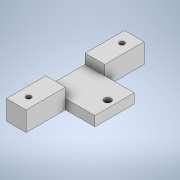
# Autodesk Inventor part: clawstack
Saved by Autodesk Inventor 2020 (Build 240168000, 168)
## iProperties
Created: 2020-03-11
Part Number: clawstack
Material: Generic
Document SubType Name: Modeling
Designer: cs1874
Density: 1 g/cm^3
Appearance: Default
Author: cs1874
Autodesk Inventor part; units mm, degrees
ref_plane "YZ Plane" through (0, 0, 0) normal (1, 0, 0) x (0, 1, 0)
ref_plane "XZ Plane" through (0, 0, 0) normal (0, 1, 0) x (-1, 0, 0)
ref_plane "XY Plane" through (0, 0, 0) normal (0, 0, 1) x (1, 0, 0)
sketch "Sketch1" plane through (0, 0, 0) normal (0, 1, 0) x (-1, 0, 0)
  line L0 (0, 0) -> (10, 0)
  line L1 (10, 0) -> (10, -60)
  line L2 (10, -60) -> (0, -60)
  line L3 (0, -60) -> (0, 0)
  line L4 (5, 0) -> (5, -6.25)
  circle A0 centre (5, -6.25) radius 1.3
  line L5 (5, -60) -> (5, -53.75)
  circle A1 centre (5, -53.75) radius 1.3
  dimension "d0" = 10
  dimension "d1" = 60
  dimension "d2" = 6.25
  dimension "d3" = 2.6
  dimension "d4" = 6.25
  dimension "d5" = 2.6
  constraints: 12 end point, 2 centre point, 2 coincident, 2 midpoint, 2 parallel, 2 vertical, 1 horizontal, 1 perpendicular
  measures "d0" distance of L1.end L2.end
  measures "d1" distance of L0.end L1.end
  measures "d2" distance of L4.start L4.end
  measures "d3" diameter of A0
  measures "d4" distance of L5.start L5.end
  measures "d5" diameter of A1
extrude "Extrusion1" add sketch "Sketch1" along normal blind 10
sketch "Sketch4" plane through (0, 10, 0) normal (0, 1, 0) x (1, 0, 0)
  line L0 (0, 0) -> (0, 60) projected
  line L1 (0, 0) -> (0, 10)
  line L2 (0, 60) -> (0, 40)
  line L3 (-10, 60) -> (-10, 0) projected
  line L4 (-10, 10) -> (-10, 50)
  line L5 (0, 50) -> (0, 10)
  line L6 (-10, 0) -> (0, 0) projected
  line L7 (0, 0) -> (0, 20)
  line L8 (0, 20) -> (-10, 20)
  line L9 (-10, 60) -> (-10, 40)
  line L10 (-10, 60) -> (10, 60) construction
  line L11 (-10, 40) -> (0, 40)
  dimension "d19" = 20
  dimension "d20" = 20
  dimension "d21" = 90
  constraints: 18 end point, 5 point on line, 3 perpendicular, 1 collinear, 1 horizontal, 1 parallel
  measures "d19" distance of L0.start L7.end
  measures "d20" distance of L3.start L9.end
  measures "d21" angle of L9 L10
extrude "Extrusion3" cut sketch "Sketch4" against normal blind 5 contours L8 L3 L11 L0
sketch "Sketch8" plane through (0, 0, 0) normal (1, 0, 0) x (0, 0, -1)
  line L0 (40, 5) -> (20, 5) projected
  line L1 (20, 5) -> (20, 0)
  line L2 (40, 5) -> (40, 0)
  line L3 (60, 0) -> (0, 0) projected
  constraints: 4 end point, 2 vertical, 1 point on line
extrude "Extrusion5" add sketch "Sketch8" along normal blind 15
sketch "Sketch9" plane through (0, 5, 0) normal (0, 1, 0) x (1, 0, 0)
  line L0 (15, 40) -> (15, 20) projected
  line L1 (15, 30) -> (11.5, 30)
  circle A0 centre (11.5, 30) radius 1.75
  point P0 (0, 0)
  dimension "d24" = 3.5
  dimension "d25" = 3.5
  constraints: 2 end point, 1 centre point, 1 coincident, 1 horizontal, 1 midpoint
  measures "d24" distance of L1.start L1.end
  measures "d25" diameter of A0
extrude "Extrusion6" cut sketch "Sketch9" against normal blind 5
body "Solid1"
